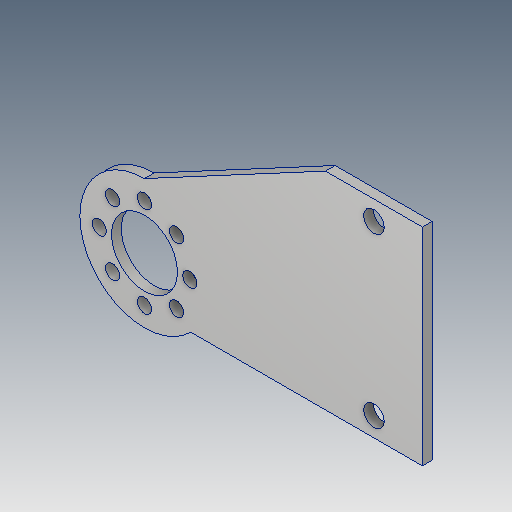
# Autodesk Inventor part: サーボ支え板A_アルミ(A2017)_t1.5
Saved by Autodesk Inventor 2019.4 (Build 234330000, 330)
## iProperties
Created: 2019-06-16
Part Number: サーボ支え板A_アルミ(A2017)_t1.5
Material: アルミニウム 6061
Document SubType Name: Modeling
Designer: 長谷川翔一
Mass: 4.89907 g
Surface Area: 28.1145 cm^2
Volume: 1.81447 cm^3
Density: 2.7 g/cm^3
Appearance: アルミニウム - フラット
Author: 長谷川翔一
Autodesk Inventor part; units mm, degrees
ref_plane "YZ Plane" through (0, 0, 0) normal (1, 0, 0) x (0, 1, 0)
ref_plane "XZ Plane" through (0, 0, 0) normal (0, 1, 0) x (-1, 0, 0)
ref_plane "XY Plane" through (0, 0, 0) normal (0, 0, 1) x (1, 0, 0)
sketch "スケッチ1" plane through (0, 0, 0) normal (0, 0, 1) x (1, 0, 0)
  arc A0 (0, 10) -> (7.1414, -7) centre (0, 0) ccw
  circle A1 centre (0, 0) radius 7 construction
  circle A2 centre (0, 7) radius 1.1
  circle A3 centre (0, 0) radius 7 construction
  circle A4 centre (-4.9497, 4.9497) radius 1.1
  circle A5 centre (0, 0) radius 7 construction
  circle A6 centre (-7, 0) radius 1.1
  circle A7 centre (0, 0) radius 7 construction
  circle A8 centre (-4.9497, -4.9497) radius 1.1
  circle A9 centre (0, 0) radius 7 construction
  circle A10 centre (0, -7) radius 1.1
  circle A11 centre (0, 0) radius 7 construction
  circle A12 centre (4.9497, -4.9497) radius 1.1
  circle A13 centre (0, 0) radius 7 construction
  circle A14 centre (7, 0) radius 1.1
  circle A15 centre (0, 0) radius 7 construction
  circle A16 centre (4.9497, 4.9497) radius 1.1
  line L0 (0, 10) -> (28, 25)
  circle A17 centre (0, 0) radius 5.1
  line L1 (43, -7) -> (43, 25)
  line L2 (7.1414, -7) -> (43, -7)
  line L3 (43, -7) -> (28, -7)
  line L4 (28, -7) -> (28, 25) construction
  line L5 (28, 25) -> (43, 25)
  line L6 (35.5, 25) -> (35.5, -7) construction
  line L7 (43, 9) -> (28, 9) construction
  circle A18 centre (35.5, 22) radius 1.6
  circle A19 centre (35.5, -4) radius 1.6
  line L8 (0, 0) -> (-10, 0) construction
  circle A20 centre (35.5, 22) radius 3 construction
  circle A21 centre (35.5, -4) radius 3 construction
  circle A22 centre (35.5, 15) radius 1.6 construction
  circle A23 centre (35.5, 15) radius 3 construction
  circle A24 centre (35.5, 3) radius 1.6 construction
  circle A25 centre (35.5, 3) radius 3 construction
  line L9 (0, 0) -> (0, 10) construction
  dimension "d1" = 14
  dimension "d0" = 20
  dimension "d2" = 2.2
  dimension "d5" = 360
  dimension "d7" = 10.2
  dimension "d11" = 15
  dimension "d12" = 90
  dimension "d13" = 3.2
  dimension "d14" = 3.2
  dimension "d15" = 35.8586
  dimension "d16" = 7
  dimension "d18" = 6
  dimension "d19" = 6
  dimension "d20" = 3.2
  dimension "d21" = 6
  dimension "d22" = 6
  dimension "d23" = 32
  constraints: 20 end point, 18 centre point, 7 coincident, 4 midpoint, 4 point on line, 3 point on circle, 2 horizontal alignment, 2 symmetric about line, 2 tangent, 2 vertical, 2 vertical alignment, 1 horizontal, 1 parallel, 1 perpendicular, 55 other
  measures "d0" diameter of A0
  measures "d2" diameter of A2
  measures "d7" diameter of A17
  measures "d11" distance of L1.start L3.end
  measures "d12" angle of L3 L4
  measures "d13" diameter of A18
  measures "d14" diameter of A19
  measures "d15" distance of L2.start L1.start
  measures "d16" distance between parallel lines of L8 L2
  measures "d18" diameter of A20
  measures "d19" diameter of A21
  measures "d20" diameter of A22
  measures "d21" diameter of A23
  measures "d22" distance from line of L7 A22.centre
  measures "d23" distance of L3.end L0.end
extrude "押し出し1" add sketch "スケッチ1" along normal blind 1.5
